Autodesk Inventor part; units mm, degrees
(part 2 of 3)
  line L233 (15.5107, -20.3284) -> (14.1645, -20.3284)
  line L234 (14.1645, -20.3284) -> (14.1645, -19.8987)
  line L235 (14.1645, -19.8987) -> (15.528, -18.3277)
  line L236 (15.528, -18.3277) -> (15.9034, -18.3277)
  line L237 (15.9034, -18.3277) -> (15.9034, -19.9999)
  line L238 (15.9034, -19.9999) -> (16.2665, -19.9999)
  line L239 (16.2665, -19.9999) -> (16.2665, -20.3284)
  line L240 (15.5107, -19.9999) -> (15.5107, -18.8094)
  line L241 (15.5107, -18.8094) -> (14.4856, -19.9999)
  line L242 (14.4856, -19.9999) -> (15.5107, -19.9999)
  line L243 (-27.5269, -31.4126) -> (-26.4993, -28.3646)
  line L244 (-26.4993, -28.3646) -> (-26.0004, -28.3646)
  line L245 (-26.0004, -28.3646) -> (-24.9729, -31.4126)
  line L246 (-24.9729, -31.4126) -> (-25.4002, -31.4126)
  line L247 (-25.4002, -31.4126) -> (-25.6768, -30.5605)
  line L248 (-25.6768, -30.5605) -> (-26.8402, -30.5605)
  line L249 (-26.8402, -30.5605) -> (-27.1168, -31.4126)
  line L250 (-27.1168, -31.4126) -> (-27.5269, -31.4126)
  line L251 (-25.788, -30.2147) -> (-26.2598, -28.7796)
  line L252 (-26.2598, -28.7796) -> (-26.7291, -30.2147)
  line L253 (-26.7291, -30.2147) -> (-25.788, -30.2147)
  line L254 (-22.9178, -31.4126) -> (-23.3031, -31.4126)
  line L255 (-23.3031, -31.4126) -> (-23.3031, -30.1085)
  spline S284 degree 2 poles (-23.3031, -30.1085) (-23.3031, -29.9504) (-23.3328, -29.6787) (-23.3772, -29.5972) knots 0 0 0 1 2 2 2
  spline S285 degree 2 poles (-23.3772, -29.5972) (-23.4242, -29.5107) (-23.5921, -29.4267) (-23.7354, -29.4267) knots 0 0 0 1 2 2 2
  spline S286 degree 2 poles (-23.7354, -29.4267) (-23.8787, -29.4267) (-24.1825, -29.5799) (-24.3282, -29.7034) knots 0 0 0 1 2 2 2
  line L256 (-24.3282, -29.7034) -> (-24.3282, -31.4126)
  line L257 (-24.3282, -31.4126) -> (-24.7135, -31.4126)
  line L258 (-24.7135, -31.4126) -> (-24.7135, -29.1254)
  line L259 (-24.7135, -29.1254) -> (-24.3282, -29.1254)
  line L260 (-24.3282, -29.1254) -> (-24.3282, -29.3798)
  spline S287 degree 2 poles (-24.3282, -29.3798) (-24.1553, -29.2242) (-23.8218, -29.0612) (-23.6341, -29.0612) knots 0 0 0 1 2 2 2
  spline S288 degree 2 poles (-23.6341, -29.0612) (-23.2982, -29.0612) (-22.9178, -29.5058) (-22.9178, -29.9281) knots 0 0 0 1 2 2 2
  line L261 (-22.9178, -29.9281) -> (-22.9178, -31.4126)
  line L262 (-20.6182, -31.4126) -> (-21.0036, -31.4126)
  line L263 (-21.0036, -31.4126) -> (-21.0036, -31.1804)
  spline S289 degree 2 poles (-21.0036, -31.1804) (-21.0925, -31.2545) (-21.2234, -31.3533) (-21.3123, -31.3953) knots 0 0 0 1 2 2 2
  spline S290 degree 2 poles (-21.3123, -31.3953) (-21.3938, -31.4349) (-21.5692, -31.4768) (-21.6853, -31.4768) knots 0 0 0 1 2 2 2
  spline S291 degree 2 poles (-21.6853, -31.4768) (-21.873, -31.4768) (-22.1892, -31.3212) (-22.3003, -31.1706) knots 0 0 0 1 2 2 2
  spline S292 degree 2 poles (-22.3003, -31.1706) (-22.4115, -31.0199) (-22.535, -30.5753) (-22.535, -30.2863) knots 0 0 0 1 2 2 2
  spline S293 degree 2 poles (-22.535, -30.2863) (-22.535, -29.985) (-22.3794, -29.5453) (-22.2435, -29.3798) knots 0 0 0 1 2 2 2
  spline S294 degree 2 poles (-22.2435, -29.3798) (-22.1175, -29.2316) (-21.7643, -29.0612) (-21.5692, -29.0612) knots 0 0 0 1 2 2 2
  spline S295 degree 2 poles (-21.5692, -29.0612) (-21.3988, -29.0612) (-21.1444, -29.1377) (-21.0036, -29.2168) knots 0 0 0 1 2 2 2
  line L264 (-21.0036, -29.2168) -> (-21.0036, -28.2288)
  line L265 (-21.0036, -28.2288) -> (-20.6182, -28.2288)
  line L266 (-20.6182, -28.2288) -> (-20.6182, -31.4126)
  line L267 (-21.0036, -30.8569) -> (-21.0036, -29.5354)
  spline S296 degree 2 poles (-21.0036, -29.5354) (-21.1468, -29.4663) (-21.3741, -29.4144) (-21.505, -29.4144) knots 0 0 0 1 2 2 2
  spline S297 degree 2 poles (-21.505, -29.4144) (-21.8014, -29.4144) (-22.1373, -29.859) (-22.1373, -30.2789) knots 0 0 0 1 2 2 2
  spline S298 degree 2 poles (-22.1373, -30.2789) (-22.1373, -30.684) (-21.8804, -31.1113) (-21.5964, -31.1113) knots 0 0 0 1 2 2 2
  spline S299 degree 2 poles (-21.5964, -31.1113) (-21.4457, -31.1113) (-21.1394, -30.973) (-21.0036, -30.8569) knots 0 0 0 1 2 2 2
  line L268 (-18.8472, -29.5379) -> (-18.867, -29.5379)
  spline S300 degree 2 poles (-18.867, -29.5379) (-18.9115, -29.5255) (-19.0078, -29.5206) (-19.0745, -29.5206) knots 0 0 0 1 2 2 2
  spline S301 degree 2 poles (-19.0745, -29.5206) (-19.2301, -29.5206) (-19.5364, -29.6564) (-19.6747, -29.7898) knots 0 0 0 1 2 2 2
  line L269 (-19.6747, -29.7898) -> (-19.6747, -31.4126)
  line L270 (-19.6747, -31.4126) -> (-20.06, -31.4126)
  line L271 (-20.06, -31.4126) -> (-20.06, -29.1254)
  line L272 (-20.06, -29.1254) -> (-19.6747, -29.1254)
  line L273 (-19.6747, -29.1254) -> (-19.6747, -29.4663)
  spline S302 degree 2 poles (-19.6747, -29.4663) (-19.4647, -29.2785) (-19.151, -29.1254) (-19.0028, -29.1254) knots 0 0 0 1 2 2 2
  spline S303 degree 2 poles (-19.0028, -29.1254) (-18.9436, -29.1254) (-18.8843, -29.1303) (-18.8472, -29.1377) knots 0 0 0 1 2 2 2
  line L274 (-18.8472, -29.1377) -> (-18.8472, -29.5379)
  spline S304 degree 2 poles (-17.5554, -31.4645) (-18.1038, -31.4645) (-18.7064, -30.8495) (-18.7064, -30.2814) knots 0 0 0 1 2 2 2
  spline S305 degree 2 poles (-18.7064, -30.2814) (-18.7064, -29.7231) (-18.1211, -29.0612) (-17.6493, -29.0612) knots 0 0 0 1 2 2 2
  spline S306 degree 2 poles (-17.6493, -29.0612) (-17.4369, -29.0612) (-17.1083, -29.1847) (-16.9873, -29.3156) knots 0 0 0 1 2 2 2
  spline S307 degree 2 poles (-16.9873, -29.3156) (-16.8638, -29.4465) (-16.7329, -29.8244) (-16.7329, -30.0986) knots 0 0 0 1 2 2 2
  line L275 (-16.7329, -30.0986) -> (-16.7329, -30.3085)
  line L276 (-16.7329, -30.3085) -> (-18.3162, -30.3085)
  spline S308 degree 2 poles (-18.3162, -30.3085) (-18.3162, -30.7062) (-17.916, -31.1286) (-17.5604, -31.1286) knots 0 0 0 1 2 2 2
  spline S309 degree 2 poles (-17.5604, -31.1286) (-17.4344, -31.1286) (-17.1899, -31.0718) (-17.0911, -31.0273) knots 0 0 0 1 2 2 2
  spline S310 degree 2 poles (-17.0911, -31.0273) (-16.9873, -30.9779) (-16.8441, -30.8915) (-16.7971, -30.8519) knots 0 0 0 1 2 2 2
  line L277 (-16.7971, -30.8519) -> (-16.7749, -30.8519)
  line L278 (-16.7749, -30.8519) -> (-16.7749, -31.2718)
  spline S311 degree 2 poles (-16.7749, -31.2718) (-16.8416, -31.299) (-17.0441, -31.378) (-17.1232, -31.4003) knots 0 0 0 1 2 2 2
  spline S312 degree 2 poles (-17.1232, -31.4003) (-17.2343, -31.4324) (-17.4171, -31.4645) (-17.5554, -31.4645) knots 0 0 0 1 2 2 2
  spline S313 degree 2 poles (-17.1083, -30.0146) (-17.1133, -29.859) (-17.1775, -29.6317) (-17.2393, -29.5552) knots 0 0 0 1 2 2 2
  spline S314 degree 2 poles (-17.2393, -29.5552) (-17.3059, -29.4687) (-17.5159, -29.3773) (-17.6715, -29.3773) knots 0 0 0 1 2 2 2
  spline S315 degree 2 poles (-17.6715, -29.3773) (-17.8246, -29.3773) (-18.0395, -29.4687) (-18.1285, -29.5576) knots 0 0 0 1 2 2 2
  spline S316 degree 2 poles (-18.1285, -29.5576) (-18.2149, -29.649) (-18.3038, -29.8689) (-18.3162, -30.0146) knots 0 0 0 1 2 2 2
  line L279 (-18.3162, -30.0146) -> (-17.1083, -30.0146)
  line L280 (-13.5713, -29.1254) -> (-14.1517, -31.4126)
  line L281 (-14.1517, -31.4126) -> (-14.5074, -31.4126)
  line L282 (-14.5074, -31.4126) -> (-15.0656, -29.649)
  line L283 (-15.0656, -29.649) -> (-15.6214, -31.4126)
  line L284 (-15.6214, -31.4126) -> (-15.9746, -31.4126)
  line L285 (-15.9746, -31.4126) -> (-16.56, -29.1254)
  line L286 (-16.56, -29.1254) -> (-16.1599, -29.1254)
  line L287 (-16.1599, -29.1254) -> (-15.7548, -30.8964)
  line L288 (-15.7548, -30.8964) -> (-15.2138, -29.1254)
  line L289 (-15.2138, -29.1254) -> (-14.8952, -29.1254)
  line L290 (-14.8952, -29.1254) -> (-14.3395, -30.8964)
  line L291 (-14.3395, -30.8964) -> (-13.9591, -29.1254)
  line L292 (-13.9591, -29.1254) -> (-13.5713, -29.1254)
  line L293 (-10.0713, -28.7253) -> (-11.4891, -28.7253)
  line L294 (-11.4891, -28.7253) -> (-11.4891, -29.5848)
  line L295 (-11.4891, -29.5848) -> (-10.1305, -29.5848)
  line L296 (-10.1305, -29.5848) -> (-10.1305, -29.9454)
  line L297 (-10.1305, -29.9454) -> (-11.4891, -29.9454)
  line L298 (-11.4891, -29.9454) -> (-11.4891, -31.4126)
  line L299 (-11.4891, -31.4126) -> (-11.8941, -31.4126)
  line L300 (-11.8941, -31.4126) -> (-11.8941, -28.3646)
  line L301 (-11.8941, -28.3646) -> (-10.0713, -28.3646)
  line L302 (-10.0713, -28.3646) -> (-10.0713, -28.7253)
  line L303 (-7.9594, -31.4126) -> (-8.3447, -31.4126)
  line L304 (-8.3447, -31.4126) -> (-8.3447, -31.1607)
  spline S317 degree 2 poles (-8.3447, -31.1607) (-8.5226, -31.3163) (-8.8412, -31.4768) (-9.0388, -31.4768) knots 0 0 0 1 2 2 2
  spline S318 degree 2 poles (-9.0388, -31.4768) (-9.187, -31.4768) (-9.4513, -31.378) (-9.5476, -31.2718) knots 0 0 0 1 2 2 2
  spline S319 degree 2 poles (-9.5476, -31.2718) (-9.6464, -31.1656) (-9.7551, -30.8421) (-9.7551, -30.6099) knots 0 0 0 1 2 2 2
  line L305 (-9.7551, -30.6099) -> (-9.7551, -29.1254)
  line L306 (-9.7551, -29.1254) -> (-9.3698, -29.1254)
  line L307 (-9.3698, -29.1254) -> (-9.3698, -30.4296)
  spline S320 degree 2 poles (-9.3698, -30.4296) (-9.3698, -30.6123) (-9.3426, -30.8519) (-9.2957, -30.9409) knots 0 0 0 1 2 2 2
  spline S321 degree 2 poles (-9.2957, -30.9409) (-9.2488, -31.0298) (-9.0882, -31.1113) (-8.9375, -31.1113) knots 0 0 0 1 2 2 2
  spline S322 degree 2 poles (-8.9375, -31.1113) (-8.7967, -31.1113) (-8.4781, -30.9507) (-8.3447, -30.8346) knots 0 0 0 1 2 2 2
  line L308 (-8.3447, -30.8346) -> (-8.3447, -29.1254)
  line L309 (-8.3447, -29.1254) -> (-7.9594, -29.1254)
  line L310 (-7.9594, -29.1254) -> (-7.9594, -31.4126)
  spline S323 degree 2 poles (-7.3197, -31.7782) (-7.2801, -31.7955) (-7.1295, -31.8498) (-7.0331, -31.8721) knots 0 0 0 1 2 2 2
  spline S324 degree 2 poles (-7.0331, -31.8721) (-6.9269, -31.8992) (-6.7466, -31.9313) (-6.6404, -31.9313) knots 0 0 0 1 2 2 2
  spline S325 degree 2 poles (-6.6404, -31.9313) (-6.4626, -31.9313) (-6.2156, -31.8375) (-6.1464, -31.7535) knots 0 0 0 1 2 2 2
  spline S326 degree 2 poles (-6.1464, -31.7535) (-6.0797, -31.6695) (-6.0279, -31.4497) (-6.0279, -31.3089) knots 0 0 0 1 2 2 2
  line L311 (-6.0279, -31.3089) -> (-6.0279, -31.1088)
  spline S327 degree 2 poles (-6.0279, -31.1088) (-6.1835, -31.2447) (-6.4823, -31.3731) (-6.7071, -31.3731) knots 0 0 0 1 2 2 2
  spline S328 degree 2 poles (-6.7071, -31.3731) (-7.0974, -31.3731) (-7.5593, -30.7927) (-7.5593, -30.2468) knots 0 0 0 1 2 2 2
  spline S329 degree 2 poles (-7.5593, -30.2468) (-7.5593, -29.9627) (-7.3987, -29.5231) (-7.2653, -29.3675) knots 0 0 0 1 2 2 2
  spline S330 degree 2 poles (-7.2653, -29.3675) (-7.1369, -29.2217) (-6.7837, -29.0612) (-6.596, -29.0612) knots 0 0 0 1 2 2 2
  spline S331 degree 2 poles (-6.596, -29.0612) (-6.4181, -29.0612) (-6.1588, -29.1452) (-6.0279, -29.2217) knots 0 0 0 1 2 2 2
  line L312 (-6.0279, -29.2217) -> (-6.0056, -29.1254)
  line L313 (-6.0056, -29.1254) -> (-5.6425, -29.1254)
  line L314 (-5.6425, -29.1254) -> (-5.6425, -31.1508)
  spline S332 degree 2 poles (-5.6425, -31.1508) (-5.6425, -31.7337) (-6.1489, -32.2771) (-6.6701, -32.2771) knots 0 0 0 1 2 2 2
  spline S333 degree 2 poles (-6.6701, -32.2771) (-6.838, -32.2771) (-7.1888, -32.2228) (-7.3394, -32.1783) knots 0 0 0 1 2 2 2
  line L315 (-7.3394, -32.1783) -> (-7.3394, -31.7782)
  line L316 (-7.3394, -31.7782) -> (-7.3197, -31.7782)
  line L317 (-6.0279, -30.7927) -> (-6.0279, -29.5354)
  spline S334 degree 2 poles (-6.0279, -29.5354) (-6.1711, -29.4663) (-6.4132, -29.407) (-6.5342, -29.407) knots 0 0 0 1 2 2 2
  spline S335 degree 2 poles (-6.5342, -29.407) (-6.8257, -29.407) (-7.1616, -29.8368) (-7.1616, -30.2394) knots 0 0 0 1 2 2 2
  spline S336 degree 2 poles (-7.1616, -30.2394) (-7.1616, -30.6198) (-6.9072, -31.0174) (-6.6207, -31.0174) knots 0 0 0 1 2 2 2
  spline S337 degree 2 poles (-6.6207, -31.0174) (-6.47, -31.0174) (-6.1538, -30.8989) (-6.0279, -30.7927) knots 0 0 0 1 2 2 2
  spline S338 degree 2 poles (-3.8098, -31.1706) (-3.8567, -31.2051) (-4.0148, -31.3286) (-4.0889, -31.3657) knots 0 0 0 1 2 2 2
  spline S339 degree 2 poles (-4.0889, -31.3657) (-4.1902, -31.42) (-4.3803, -31.4768) (-4.5533, -31.4768) knots 0 0 0 1 2 2 2
  spline S340 degree 2 poles (-4.5533, -31.4768) (-4.694, -31.4768) (-4.9485, -31.3706) (-5.0448, -31.2743) knots 0 0 0 1 2 2 2
  spline S341 degree 2 poles (-5.0448, -31.2743) (-5.1362, -31.1804) (-5.2473, -30.9038) (-5.2473, -30.7507) knots 0 0 0 1 2 2 2
  spline S342 degree 2 poles (-5.2473, -30.7507) (-5.2473, -30.5135) (-5.0473, -30.1776) (-4.8299, -30.0813) knots 0 0 0 1 2 2 2
  spline S343 degree 2 poles (-4.8299, -30.0813) (-4.6372, -29.9924) (-4.1136, -29.9257) (-3.8098, -29.9084) knots 0 0 0 1 2 2 2
  line L318 (-3.8098, -29.9084) -> (-3.8098, -29.8343)
  spline S344 degree 2 poles (-3.8098, -29.8343) (-3.8098, -29.7009) (-3.8913, -29.5354) (-3.9654, -29.4885) knots 0 0 0 1 2 2 2
  spline S345 degree 2 poles (-3.9654, -29.4885) (-4.0395, -29.4416) (-4.2519, -29.4119) (-4.3655, -29.4119) knots 0 0 0 1 2 2 2
  spline S346 degree 2 poles (-4.3655, -29.4119) (-4.4989, -29.4119) (-4.8595, -29.491) (-5.0398, -29.5675) knots 0 0 0 1 2 2 2
  line L319 (-5.0398, -29.5675) -> (-5.0621, -29.5675)
  line L320 (-5.0621, -29.5675) -> (-5.0621, -29.1748)
  spline S347 degree 2 poles (-5.0621, -29.1748) (-4.9559, -29.1452) (-4.5582, -29.0711) (-4.3631, -29.0711) knots 0 0 0 1 2 2 2
  spline S348 degree 2 poles (-4.3631, -29.0711) (-4.1259, -29.0711) (-3.8024, -29.1452) (-3.6739, -29.2415) knots 0 0 0 1 2 2 2
  spline S349 degree 2 poles (-3.6739, -29.2415) (-3.548, -29.3353) (-3.4245, -29.6342) (-3.4245, -29.8491) knots 0 0 0 1 2 2 2
  line L321 (-3.4245, -29.8491) -> (-3.4245, -31.4126)
  line L322 (-3.4245, -31.4126) -> (-3.8098, -31.4126)
  line L323 (-3.8098, -31.4126) -> (-3.8098, -31.1706)
  line L324 (-3.8098, -30.8495) -> (-3.8098, -30.2147)
  spline S350 degree 2 poles (-3.8098, -30.2147) (-3.9481, -30.227) (-4.3655, -30.269) (-4.4964, -30.3085) knots 0 0 0 1 2 2 2
  spline S351 degree 2 poles (-4.4964, -30.3085) (-4.6496, -30.3555) (-4.8497, -30.5506) (-4.8497, -30.7235) knots 0 0 0 1 2 2 2
  spline S352 degree 2 poles (-4.8497, -30.7235) (-4.8497, -30.9211) (-4.6274, -31.1212) (-4.4149, -31.1212) knots 0 0 0 1 2 2 2
  spline S353 degree 2 poles (-4.4149, -31.1212) (-4.2346, -31.1212) (-3.9382, -30.9656) (-3.8098, -30.8495) knots 0 0 0 1 2 2 2
  spline S354 degree 2 poles (-2.1919, -31.4571) (-2.5056, -31.4571) (-2.8588, -31.0989) (-2.8588, -30.7111) knots 0 0 0 1 2 2 2
  line L325 (-2.8588, -30.7111) -> (-2.8588, -29.444)
  line L326 (-2.8588, -29.444) -> (-3.1182, -29.444)
  line L327 (-3.1182, -29.444) -> (-3.1182, -29.1254)
  line L328 (-3.1182, -29.1254) -> (-2.8588, -29.1254)
  line L329 (-2.8588, -29.1254) -> (-2.8588, -28.4684)
  line L330 (-2.8588, -28.4684) -> (-2.4735, -28.4684)
  line L331 (-2.4735, -28.4684) -> (-2.4735, -29.1254)
  line L332 (-2.4735, -29.1254) -> (-1.7646, -29.1254)
  line L333 (-1.7646, -29.1254) -> (-1.7646, -29.444)
  line L334 (-1.7646, -29.444) -> (-2.4735, -29.444)
  line L335 (-2.4735, -29.444) -> (-2.4735, -30.5333)
  spline S355 degree 2 poles (-2.4735, -30.5333) (-2.4735, -30.7062) (-2.4611, -30.8964) (-2.4192, -30.9779) knots 0 0 0 1 2 2 2
  spline S356 degree 2 poles (-2.4192, -30.9779) (-2.3846, -31.0495) (-2.229, -31.1212) (-2.0956, -31.1212) knots 0 0 0 1 2 2 2
  spline S357 degree 2 poles (-2.0956, -31.1212) (-2.0017, -31.1212) (-1.8264, -31.0644) (-1.7868, -31.0471) knots 0 0 0 1 2 2 2
  line L336 (-1.7868, -31.0471) -> (-1.7646, -31.0471)
  line L337 (-1.7646, -31.0471) -> (-1.7646, -31.3929)
  spline S358 degree 2 poles (-1.7646, -31.3929) (-1.8733, -31.4225) (-2.0956, -31.4571) (-2.1919, -31.4571) knots 0 0 0 1 2 2 2
  spline S359 degree 2 poles (-0.4876, -31.4645) (-1.0359, -31.4645) (-1.6386, -30.8495) (-1.6386, -30.2814) knots 0 0 0 1 2 2 2
  spline S360 degree 2 poles (-1.6386, -30.2814) (-1.6386, -29.7231) (-1.0532, -29.0612) (-0.5815, -29.0612) knots 0 0 0 1 2 2 2
  spline S361 degree 2 poles (-0.5815, -29.0612) (-0.369, -29.0612) (-0.0405, -29.1847) (0.0805, -29.3156) knots 0 0 0 1 2 2 2
  spline S362 degree 2 poles (0.0805, -29.3156) (0.204, -29.4465) (0.3349, -29.8244) (0.3349, -30.0986) knots 0 0 0 1 2 2 2
  line L338 (0.3349, -30.0986) -> (0.3349, -30.3085)
  line L339 (0.3349, -30.3085) -> (-1.2484, -30.3085)
  spline S363 degree 2 poles (-1.2484, -30.3085) (-1.2484, -30.7062) (-0.8482, -31.1286) (-0.4925, -31.1286) knots 0 0 0 1 2 2 2
  spline S364 degree 2 poles (-0.4925, -31.1286) (-0.3666, -31.1286) (-0.122, -31.0718) (-0.0232, -31.0273) knots 0 0 0 1 2 2 2
  spline S365 degree 2 poles (-0.0232, -31.0273) (0.0805, -30.9779) (0.2238, -30.8915) (0.2707, -30.8519) knots 0 0 0 1 2 2 2
  line L340 (0.2707, -30.8519) -> (0.2929, -30.8519)
  line L341 (0.2929, -30.8519) -> (0.2929, -31.2718)
  spline S366 degree 2 poles (0.2929, -31.2718) (0.2262, -31.299) (0.0237, -31.378) (-0.0554, -31.4003) knots 0 0 0 1 2 2 2
  spline S367 degree 2 poles (-0.0554, -31.4003) (-0.1665, -31.4324) (-0.3493, -31.4645) (-0.4876, -31.4645) knots 0 0 0 1 2 2 2
  spline S368 degree 2 poles (-0.0405, -30.0146) (-0.0455, -29.859) (-0.1097, -29.6317) (-0.1714, -29.5552) knots 0 0 0 1 2 2 2
  spline S369 degree 2 poles (-0.1714, -29.5552) (-0.2381, -29.4687) (-0.4481, -29.3773) (-0.6037, -29.3773) knots 0 0 0 1 2 2 2
  spline S370 degree 2 poles (-0.6037, -29.3773) (-0.7568, -29.3773) (-0.9717, -29.4687) (-1.0606, -29.5576) knots 0 0 0 1 2 2 2
  spline S371 degree 2 poles (-1.0606, -29.5576) (-1.1471, -29.649) (-1.236, -29.8689) (-1.2484, -30.0146) knots 0 0 0 1 2 2 2
  line L342 (-1.2484, -30.0146) -> (-0.0405, -30.0146)
  line L343 (3.0939, -30.2641) -> (1.9404, -30.2641)
  line L344 (1.9404, -30.2641) -> (1.9404, -29.8936)
  line L345 (1.9404, -29.8936) -> (3.0939, -29.8936)
  line L346 (3.0939, -29.8936) -> (3.0939, -30.2641)
  line L347 (4.566, -31.4126) -> (5.5936, -28.3646)
  line L348 (5.5936, -28.3646) -> (6.0925, -28.3646)
  line L349 (6.0925, -28.3646) -> (7.12, -31.4126)
  line L350 (7.12, -31.4126) -> (6.6927, -31.4126)
  line L351 (6.6927, -31.4126) -> (6.4161, -30.5605)
  line L352 (6.4161, -30.5605) -> (5.2527, -30.5605)
  line L353 (5.2527, -30.5605) -> (4.9761, -31.4126)
  line L354 (4.9761, -31.4126) -> (4.566, -31.4126)
  line L355 (6.3049, -30.2147) -> (5.8332, -28.7796)
  line L356 (5.8332, -28.7796) -> (5.3639, -30.2147)
  line L357 (5.3639, -30.2147) -> (6.3049, -30.2147)
  line L358 (7.7721, -31.4126) -> (7.3868, -31.4126)
  line L359 (7.3868, -31.4126) -> (7.3868, -28.2288)
  line L360 (7.3868, -28.2288) -> (7.7721, -28.2288)
  line L361 (7.7721, -28.2288) -> (7.7721, -31.4126)
  spline S372 degree 2 poles (9.3307, -31.4645) (8.7824, -31.4645) (8.1797, -30.8495) (8.1797, -30.2814) knots 0 0 0 1 2 2 2
  spline S373 degree 2 poles (8.1797, -30.2814) (8.1797, -29.7231) (8.7651, -29.0612) (9.2368, -29.0612) knots 0 0 0 1 2 2 2
  spline S374 degree 2 poles (9.2368, -29.0612) (9.4493, -29.0612) (9.7778, -29.1847) (9.8988, -29.3156) knots 0 0 0 1 2 2 2
  spline S375 degree 2 poles (9.8988, -29.3156) (10.0223, -29.4465) (10.1532, -29.8244) (10.1532, -30.0986) knots 0 0 0 1 2 2 2
  line L362 (10.1532, -30.0986) -> (10.1532, -30.3085)
  line L363 (10.1532, -30.3085) -> (8.5699, -30.3085)
  spline S376 degree 2 poles (8.5699, -30.3085) (8.5699, -30.7062) (8.9701, -31.1286) (9.3258, -31.1286) knots 0 0 0 1 2 2 2
  spline S377 degree 2 poles (9.3258, -31.1286) (9.4517, -31.1286) (9.6963, -31.0718) (9.7951, -31.0273) knots 0 0 0 1 2 2 2
  spline S378 degree 2 poles (9.7951, -31.0273) (9.8988, -30.9779) (10.0421, -30.8915) (10.089, -30.8519) knots 0 0 0 1 2 2 2
  line L364 (10.089, -30.8519) -> (10.1112, -30.8519)
  line L365 (10.1112, -30.8519) -> (10.1112, -31.2718)
  spline S379 degree 2 poles (10.1112, -31.2718) (10.0445, -31.299) (9.842, -31.378) (9.763, -31.4003) knots 0 0 0 1 2 2 2
  spline S380 degree 2 poles (9.763, -31.4003) (9.6518, -31.4324) (9.469, -31.4645) (9.3307, -31.4645) knots 0 0 0 1 2 2 2
  spline S381 degree 2 poles (9.7778, -30.0146) (9.7728, -29.859) (9.7086, -29.6317) (9.6469, -29.5552) knots 0 0 0 1 2 2 2
  spline S382 degree 2 poles (9.6469, -29.5552) (9.5802, -29.4687) (9.3702, -29.3773) (9.2146, -29.3773) knots 0 0 0 1 2 2 2
  spline S383 degree 2 poles (9.2146, -29.3773) (9.0615, -29.3773) (8.8466, -29.4687) (8.7577, -29.5576) knots 0 0 0 1 2 2 2
  spline S384 degree 2 poles (8.7577, -29.5576) (8.6712, -29.649) (8.5823, -29.8689) (8.5699, -30.0146) knots 0 0 0 1 2 2 2
  line L366 (8.5699, -30.0146) -> (9.7778, -30.0146)
  spline S385 degree 2 poles (11.4525, -31.4645) (11.2153, -31.4645) (10.8226, -31.3188) (10.6818, -31.1706) knots 0 0 0 1 2 2 2
  spline S386 degree 2 poles (10.6818, -31.1706) (10.541, -31.0248) (10.3854, -30.5753) (10.3854, -30.274) knots 0 0 0 1 2 2 2
  spline S387 degree 2 poles (10.3854, -30.274) (10.3854, -29.9726) (10.546, -29.5329) (10.6818, -29.3847) knots 0 0 0 1 2 2 2
  spline S388 degree 2 poles (10.6818, -29.3847) (10.8177, -29.2341) (11.2203, -29.0735) (11.4525, -29.0735) knots 0 0 0 1 2 2 2
  spline S389 degree 2 poles (11.4525, -29.0735) (11.6402, -29.0735) (11.9909, -29.1797) (12.1268, -29.2489) knots 0 0 0 1 2 2 2
  line L367 (12.1268, -29.2489) -> (12.1268, -29.6811)
  line L368 (12.1268, -29.6811) -> (12.1045, -29.6811)
  spline S390 degree 2 poles (12.1045, -29.6811) (12.0625, -29.6466) (11.9341, -29.5576) (11.8427, -29.5107) knots 0 0 0 1 2 2 2
  spline S391 degree 2 poles (11.8427, -29.5107) (11.7612, -29.4712) (11.5438, -29.4094) (11.445, -29.4094) knots 0 0 0 1 2 2 2
  spline S392 degree 2 poles (11.445, -29.4094) (11.1462, -29.4094) (10.7831, -29.8615) (10.7831, -30.274) knots 0 0 0 1 2 2 2
  spline S393 degree 2 poles (10.7831, -30.274) (10.7831, -30.6766) (11.1338, -31.1286) (11.445, -31.1286) knots 0 0 0 1 2 2 2
  spline S394 degree 2 poles (11.445, -31.1286) (11.6328, -31.1286) (11.9736, -30.973) (12.1045, -30.8519) knots 0 0 0 1 2 2 2
  line L369 (12.1045, -30.8519) -> (12.1268, -30.8519)
  line L370 (12.1268, -30.8519) -> (12.1268, -31.2842)
  spline S395 degree 2 poles (12.1268, -31.2842) (12.07, -31.3114) (11.8971, -31.3879) (11.8279, -31.4052) knots 0 0 0 1 2 2 2
  spline S396 degree 2 poles (11.8279, -31.4052) (11.7291, -31.4349) (11.5735, -31.4645) (11.4525, -31.4645) knots 0 0 0 1 2 2 2
  spline S397 degree 2 poles (16.2196, -29.8911) (16.2196, -30.3085) (15.8812, -30.9804) (15.5971, -31.1681) knots 0 0 0 1 2 2 2
  spline S398 degree 2 poles (15.5971, -31.1681) (15.365, -31.3138) (14.8882, -31.4126) (14.5177, -31.4126) knots 0 0 0 1 2 2 2
  line L371 (14.5177, -31.4126) -> (13.8163, -31.4126)
  line L372 (13.8163, -31.4126) -> (13.8163, -28.3646)
  line L373 (13.8163, -28.3646) -> (14.5103, -28.3646)
  spline S399 degree 2 poles (14.5103, -28.3646) (14.9401, -28.3646) (15.4292, -28.4931) (15.6021, -28.6067) knots 0 0 0 1 2 2 2
  spline S400 degree 2 poles (15.6021, -28.6067) (15.896, -28.8018) (16.2196, -29.4465) (16.2196, -29.8911) knots 0 0 0 1 2 2 2
  spline S401 degree 2 poles (15.7972, -29.8862) (15.7972, -29.5354) (15.565, -29.0389) (15.3353, -28.8982) knots 0 0 0 1 2 2 2
  spline S402 degree 2 poles (15.3353, -28.8982) (15.1723, -28.8018) (14.8043, -28.7154) (14.5301, -28.7154) knots 0 0 0 1 2 2 2
  line L374 (14.5301, -28.7154) -> (14.2213, -28.7154)
  line L375 (14.2213, -28.7154) -> (14.2213, -31.0619)
  line L376 (14.2213, -31.0619) -> (14.5301, -31.0619)
  spline S403 degree 2 poles (14.5301, -31.0619) (14.7993, -31.0619) (15.2069, -30.9754) (15.3724, -30.8593) knots 0 0 0 1 2 2 2
  spline S404 degree 2 poles (15.3724, -30.8593) (15.5848, -30.7161) (15.7972, -30.2418) (15.7972, -29.8862) knots 0 0 0 1 2 2 2
  spline S405 degree 2 poles (17.9041, -31.1706) (17.8572, -31.2051) (17.6991, -31.3286) (17.625, -31.3657) knots 0 0 0 1 2 2 2
  spline S406 degree 2 poles (17.625, -31.3657) (17.5238, -31.42) (17.3336, -31.4768) (17.1607, -31.4768) knots 0 0 0 1 2 2 2
  spline S407 degree 2 poles (17.1607, -31.4768) (17.0199, -31.4768) (16.7655, -31.3706) (16.6691, -31.2743) knots 0 0 0 1 2 2 2
  spline S408 degree 2 poles (16.6691, -31.2743) (16.5777, -31.1804) (16.4666, -30.9038) (16.4666, -30.7507) knots 0 0 0 1 2 2 2
  spline S409 degree 2 poles (16.4666, -30.7507) (16.4666, -30.5135) (16.6667, -30.1776) (16.884, -30.0813) knots 0 0 0 1 2 2 2
  spline S410 degree 2 poles (16.884, -30.0813) (17.0767, -29.9924) (17.6003, -29.9257) (17.9041, -29.9084) knots 0 0 0 1 2 2 2
  line L377 (17.9041, -29.9084) -> (17.9041, -29.8343)
  spline S411 degree 2 poles (17.9041, -29.8343) (17.9041, -29.7009) (17.8226, -29.5354) (17.7485, -29.4885) knots 0 0 0 1 2 2 2
  spline S412 degree 2 poles (17.7485, -29.4885) (17.6744, -29.4416) (17.462, -29.4119) (17.3484, -29.4119) knots 0 0 0 1 2 2 2
  spline S413 degree 2 poles (17.3484, -29.4119) (17.215, -29.4119) (16.8544, -29.491) (16.6741, -29.5675) knots 0 0 0 1 2 2 2
  line L378 (16.6741, -29.5675) -> (16.6518, -29.5675)
  line L379 (16.6518, -29.5675) -> (16.6518, -29.1748)
  spline S414 degree 2 poles (16.6518, -29.1748) (16.758, -29.1452) (17.1557, -29.0711) (17.3509, -29.0711) knots 0 0 0 1 2 2 2
  spline S415 degree 2 poles (17.3509, -29.0711) (17.588, -29.0711) (17.9115, -29.1452) (18.04, -29.2415) knots 0 0 0 1 2 2 2
  spline S416 degree 2 poles (18.04, -29.2415) (18.166, -29.3353) (18.2895, -29.6342) (18.2895, -29.8491) knots 0 0 0 1 2 2 2
  line L380 (18.2895, -29.8491) -> (18.2895, -31.4126)
  line L381 (18.2895, -31.4126) -> (17.9041, -31.4126)
  line L382 (17.9041, -31.4126) -> (17.9041, -31.1706)
  line L383 (17.9041, -30.8495) -> (17.9041, -30.2147)
  spline S417 degree 2 poles (17.9041, -30.2147) (17.7658, -30.227) (17.3484, -30.269) (17.2175, -30.3085) knots 0 0 0 1 2 2 2
  spline S418 degree 2 poles (17.2175, -30.3085) (17.0643, -30.3555) (16.8643, -30.5506) (16.8643, -30.7235) knots 0 0 0 1 2 2 2
  spline S419 degree 2 poles (16.8643, -30.7235) (16.8643, -30.9211) (17.0866, -31.1212) (17.299, -31.1212) knots 0 0 0 1 2 2 2
  spline S420 degree 2 poles (17.299, -31.1212) (17.4793, -31.1212) (17.7757, -30.9656) (17.9041, -30.8495) knots 0 0 0 1 2 2 2
  line L384 (21.4239, -31.4126) -> (21.4239, -30.0887)
  spline S421 degree 2 poles (21.4239, -30.0887) (21.4239, -29.9306) (21.3992, -29.6614) (21.3597, -29.5873) knots 0 0 0 1 2 2 2
  spline S422 degree 2 poles (21.3597, -29.5873) (21.3202, -29.5058) (21.1695, -29.4267) (21.0386, -29.4267) knots 0 0 0 1 2 2 2
  spline S423 degree 2 poles (21.0386, -29.4267) (20.92, -29.4267) (20.6483, -29.5725) (20.5051, -29.7108) knots 0 0 0 1 2 2 2
  spline S424 degree 2 poles (20.5051, -29.7108) (20.5075, -29.7454) (20.5125, -29.8417) (20.5125, -29.9059) knots 0 0 0 1 2 2 2
  line L385 (20.5125, -29.9059) -> (20.5125, -31.4126)
  line L386 (20.5125, -31.4126) -> (20.1272, -31.4126)
  line L387 (20.1272, -31.4126) -> (20.1272, -30.0887)
  spline S425 degree 2 poles (20.1272, -30.0887) (20.1272, -29.9306) (20.1025, -29.6614) (20.0629, -29.5873) knots 0 0 0 1 2 2 2
  spline S426 degree 2 poles (20.0629, -29.5873) (20.0234, -29.5058) (19.8727, -29.4267) (19.7418, -29.4267) knots 0 0 0 1 2 2 2
  spline S427 degree 2 poles (19.7418, -29.4267) (19.6183, -29.4267) (19.3442, -29.5823) (19.2157, -29.7034) knots 0 0 0 1 2 2 2
  line L388 (19.2157, -29.7034) -> (19.2157, -31.4126)
  line L389 (19.2157, -31.4126) -> (18.8304, -31.4126)
  line L390 (18.8304, -31.4126) -> (18.8304, -29.1254)
  line L391 (18.8304, -29.1254) -> (19.2157, -29.1254)
  line L392 (19.2157, -29.1254) -> (19.2157, -29.3773)
  spline S428 degree 2 poles (19.2157, -29.3773) (19.3664, -29.2267) (19.6628, -29.0612) (19.8406, -29.0612) knots 0 0 0 1 2 2 2
  spline S429 degree 2 poles (19.8406, -29.0612) (20.0432, -29.0612) (20.3569, -29.2464) (20.4384, -29.4564) knots 0 0 0 1 2 2 2
  spline S430 degree 2 poles (20.4384, -29.4564) (20.6137, -29.2612) (20.9447, -29.0612) (21.1374, -29.0612) knots 0 0 0 1 2 2 2
  spline S431 degree 2 poles (21.1374, -29.0612) (21.2856, -29.0612) (21.5277, -29.1526) (21.6166, -29.2563) knots 0 0 0 1 2 2 2
  spline S432 degree 2 poles (21.6166, -29.2563) (21.708, -29.36) (21.8092, -29.6713) (21.8092, -29.9059) knots 0 0 0 1 2 2 2
  line L393 (21.8092, -29.9059) -> (21.8092, -31.4126)
  line L394 (21.8092, -31.4126) -> (21.4239, -31.4126)
  line L395 (22.7429, -31.4126) -> (22.3576, -31.4126)
  line L396 (22.3576, -31.4126) -> (22.3576, -29.1254)
  line L397 (22.3576, -29.1254) -> (22.7429, -29.1254)
  line L398 (22.7429, -29.1254) -> (22.7429, -31.4126)
  line L399 (22.7701, -28.745) -> (22.3329, -28.745)
  line L400 (22.3329, -28.745) -> (22.3329, -28.3449)
  line L401 (22.3329, -28.3449) -> (22.7701, -28.3449)
  line L402 (22.7701, -28.3449) -> (22.7701, -28.745)
  spline S433 degree 2 poles (24.3015, -31.4645) (23.7531, -31.4645) (23.1505, -30.8495) (23.1505, -30.2814) knots 0 0 0 1 2 2 2
  spline S434 degree 2 poles (23.1505, -30.2814) (23.1505, -29.7231) (23.7358, -29.0612) (24.2076, -29.0612) knots 0 0 0 1 2 2 2
  spline S435 degree 2 poles (24.2076, -29.0612) (24.42, -29.0612) (24.7486, -29.1847) (24.8696, -29.3156) knots 0 0 0 1 2 2 2
  spline S436 degree 2 poles (24.8696, -29.3156) (24.9931, -29.4465) (25.124, -29.8244) (25.124, -30.0986) knots 0 0 0 1 2 2 2
  line L403 (25.124, -30.0986) -> (25.124, -30.3085)
  line L404 (25.124, -30.3085) -> (23.5407, -30.3085)
  spline S437 degree 2 poles (23.5407, -30.3085) (23.5407, -30.7062) (23.9409, -31.1286) (24.2965, -31.1286) knots 0 0 0 1 2 2 2
  spline S438 degree 2 poles (24.2965, -31.1286) (24.4225, -31.1286) (24.667, -31.0718) (24.7658, -31.0273) knots 0 0 0 1 2 2 2
  spline S439 degree 2 poles (24.7658, -31.0273) (24.8696, -30.9779) (25.0128, -30.8915) (25.0598, -30.8519) knots 0 0 0 1 2 2 2
  line L405 (25.0598, -30.8519) -> (25.082, -30.8519)
  line L406 (25.082, -30.8519) -> (25.082, -31.2718)
  spline S440 degree 2 poles (25.082, -31.2718) (25.0153, -31.299) (24.8128, -31.378) (24.7337, -31.4003) knots 0 0 0 1 2 2 2
  spline S441 degree 2 poles (24.7337, -31.4003) (24.6226, -31.4324) (24.4398, -31.4645) (24.3015, -31.4645) knots 0 0 0 1 2 2 2
  spline S442 degree 2 poles (24.7486, -30.0146) (24.7436, -29.859) (24.6794, -29.6317) (24.6176, -29.5552) knots 0 0 0 1 2 2 2
  spline S443 degree 2 poles (24.6176, -29.5552) (24.551, -29.4687) (24.341, -29.3773) (24.1854, -29.3773) knots 0 0 0 1 2 2 2
  spline S444 degree 2 poles (24.1854, -29.3773) (24.0322, -29.3773) (23.8174, -29.4687) (23.7284, -29.5576) knots 0 0 0 1 2 2 2
  spline S445 degree 2 poles (23.7284, -29.5576) (23.642, -29.649) (23.5531, -29.8689) (23.5407, -30.0146) knots 0 0 0 1 2 2 2
  line L407 (23.5407, -30.0146) -> (24.7486, -30.0146)
  line L408 (27.31, -31.4126) -> (26.9246, -31.4126)
  line L409 (26.9246, -31.4126) -> (26.9246, -30.1085)
  spline S446 degree 2 poles (26.9246, -30.1085) (26.9246, -29.9504) (26.895, -29.6787) (26.8505, -29.5972) knots 0 0 0 1 2 2 2
  spline S447 degree 2 poles (26.8505, -29.5972) (26.8036, -29.5107) (26.6356, -29.4267) (26.4924, -29.4267) knots 0 0 0 1 2 2 2
  spline S448 degree 2 poles (26.4924, -29.4267) (26.3491, -29.4267) (26.0453, -29.5799) (25.8996, -29.7034) knots 0 0 0 1 2 2 2
  line L410 (25.8996, -29.7034) -> (25.8996, -31.4126)
  line L411 (25.8996, -31.4126) -> (25.5143, -31.4126)
  line L412 (25.5143, -31.4126) -> (25.5143, -29.1254)
  line L413 (25.5143, -29.1254) -> (25.8996, -29.1254)
  line L414 (25.8996, -29.1254) -> (25.8996, -29.3798)
  spline S449 degree 2 poles (25.8996, -29.3798) (26.0725, -29.2242) (26.4059, -29.0612) (26.5937, -29.0612) knots 0 0 0 1 2 2 2
  spline S450 degree 2 poles (26.5937, -29.0612) (26.9296, -29.0612) (27.31, -29.5058) (27.31, -29.9281) knots 0 0 0 1 2 2 2
  line L415 (27.31, -29.9281) -> (27.31, -31.4126)
  line L416 (-24.406, -33.3831) -> (-25.436, -35.0825)
  line L417 (-25.436, -35.0825) -> (-25.436, -36.4311)
  line L418 (-25.436, -36.4311) -> (-25.8411, -36.4311)
  line L419 (-25.8411, -36.4311) -> (-25.8411, -35.1244)
  line L420 (-25.8411, -35.1244) -> (-26.8711, -33.3831)
  line L421 (-26.8711, -33.3831) -> (-26.4215, -33.3831)
  line L422 (-26.4215, -33.3831) -> (-25.6361, -34.7243)
  line L423 (-25.6361, -34.7243) -> (-24.8358, -33.3831)
  line L424 (-24.8358, -33.3831) -> (-24.406, -33.3831)
  line L425 (-22.3584, -34.1438) -> (-23.2204, -36.4311)
  line L426 (-23.2204, -36.4311) -> (-23.5662, -36.4311)
  line L427 (-23.5662, -36.4311) -> (-24.4208, -34.1438)
  line L428 (-24.4208, -34.1438) -> (-24.0034, -34.1438)
  line L429 (-24.0034, -34.1438) -> (-23.3785, -35.905)
  line L430 (-23.3785, -35.905) -> (-22.7585, -34.1438)
  line L431 (-22.7585, -34.1438) -> (-22.3584, -34.1438)
  spline S451 degree 2 poles (-20.7924, -36.189) (-20.8393, -36.2236) (-20.9974, -36.3471) (-21.0715, -36.3841) knots 0 0 0 1 2 2 2
  spline S452 degree 2 poles (-21.0715, -36.3841) (-21.1728, -36.4385) (-21.3629, -36.4953) (-21.5358, -36.4953) knots 0 0 0 1 2 2 2
  spline S453 degree 2 poles (-21.5358, -36.4953) (-21.6766, -36.4953) (-21.9311, -36.3891) (-22.0274, -36.2928) knots 0 0 0 1 2 2 2
  spline S454 degree 2 poles (-22.0274, -36.2928) (-22.1188, -36.1989) (-22.2299, -35.9223) (-22.2299, -35.7691) knots 0 0 0 1 2 2 2
  spline S455 degree 2 poles (-22.2299, -35.7691) (-22.2299, -35.532) (-22.0299, -35.1961) (-21.8125, -35.0997) knots 0 0 0 1 2 2 2
  spline S456 degree 2 poles (-21.8125, -35.0997) (-21.6198, -35.0108) (-21.0962, -34.9441) (-20.7924, -34.9268) knots 0 0 0 1 2 2 2
  line L432 (-20.7924, -34.9268) -> (-20.7924, -34.8527)
  spline S457 degree 2 poles (-20.7924, -34.8527) (-20.7924, -34.7194) (-20.8739, -34.5539) (-20.948, -34.5069) knots 0 0 0 1 2 2 2
  spline S458 degree 2 poles (-20.948, -34.5069) (-21.0221, -34.46) (-21.2345, -34.4304) (-21.3481, -34.4304) knots 0 0 0 1 2 2 2
  spline S459 degree 2 poles (-21.3481, -34.4304) (-21.4815, -34.4304) (-21.8421, -34.5094) (-22.0224, -34.586) knots 0 0 0 1 2 2 2
  line L433 (-22.0224, -34.586) -> (-22.0447, -34.586)
  line L434 (-22.0447, -34.586) -> (-22.0447, -34.1932)
  spline S460 degree 2 poles (-22.0447, -34.1932) (-21.9385, -34.1636) (-21.5408, -34.0895) (-21.3457, -34.0895) knots 0 0 0 1 2 2 2
  spline S461 degree 2 poles (-21.3457, -34.0895) (-21.1085, -34.0895) (-20.785, -34.1636) (-20.6565, -34.2599) knots 0 0 0 1 2 2 2
  spline S462 degree 2 poles (-20.6565, -34.2599) (-20.5306, -34.3538) (-20.4071, -34.6527) (-20.4071, -34.8676) knots 0 0 0 1 2 2 2
  line L435 (-20.4071, -34.8676) -> (-20.4071, -36.4311)
  line L436 (-20.4071, -36.4311) -> (-20.7924, -36.4311)
  line L437 (-20.7924, -36.4311) -> (-20.7924, -36.189)
  line L438 (-20.7924, -35.8679) -> (-20.7924, -35.2331)
  spline S463 degree 2 poles (-20.7924, -35.2331) (-20.9307, -35.2455) (-21.3481, -35.2875) (-21.479, -35.327) knots 0 0 0 1 2 2 2
  spline S464 degree 2 poles (-21.479, -35.327) (-21.6322, -35.3739) (-21.8322, -35.569) (-21.8322, -35.7419) knots 0 0 0 1 2 2 2
  spline S465 degree 2 poles (-21.8322, -35.7419) (-21.8322, -35.9395) (-21.6099, -36.1396) (-21.3975, -36.1396) knots 0 0 0 1 2 2 2
  spline S466 degree 2 poles (-21.3975, -36.1396) (-21.2172, -36.1396) (-20.9208, -35.984) (-20.7924, -35.8679) knots 0 0 0 1 2 2 2
  line L439 (-18.0704, -36.4311) -> (-18.4557, -36.4311)
  line L440 (-18.4557, -36.4311) -> (-18.4557, -35.1269)
  spline S467 degree 2 poles (-18.4557, -35.1269) (-18.4557, -34.9688) (-18.4854, -34.6971) (-18.5298, -34.6156) knots 0 0 0 1 2 2 2
  spline S468 degree 2 poles (-18.5298, -34.6156) (-18.5768, -34.5292) (-18.7447, -34.4452) (-18.888, -34.4452) knots 0 0 0 1 2 2 2
  spline S469 degree 2 poles (-18.888, -34.4452) (-19.0313, -34.4452) (-19.3351, -34.5983) (-19.4808, -34.7218) knots 0 0 0 1 2 2 2
  line L441 (-19.4808, -34.7218) -> (-19.4808, -36.4311)
  line L442 (-19.4808, -36.4311) -> (-19.8661, -36.4311)
  line L443 (-19.8661, -36.4311) -> (-19.8661, -34.1438)
  line L444 (-19.8661, -34.1438) -> (-19.4808, -34.1438)
  line L445 (-19.4808, -34.1438) -> (-19.4808, -34.3983)
  spline S470 degree 2 poles (-19.4808, -34.3983) (-19.3079, -34.2426) (-18.9744, -34.0796) (-18.7867, -34.0796) knots 0 0 0 1 2 2 2
  spline S471 degree 2 poles (-18.7867, -34.0796) (-18.4508, -34.0796) (-18.0704, -34.5242) (-18.0704, -34.9466) knots 0 0 0 1 2 2 2
  line L446 (-18.0704, -34.9466) -> (-18.0704, -36.4311)
  spline S472 degree 2 poles (-14.2641, -34.3019) (-14.2641, -34.4995) (-14.4049, -34.8552) (-14.5309, -34.9787) knots 0 0 0 1 2 2 2
  spline S473 degree 2 poles (-14.5309, -34.9787) (-14.689, -35.1343) (-15.1163, -35.2949) (-15.4423, -35.2949) knots 0 0 0 1 2 2 2
  line L447 (-15.4423, -35.2949) -> (-15.7856, -35.2949)
  line L448 (-15.7856, -35.2949) -> (-15.7856, -36.4311)
  line L449 (-15.7856, -36.4311) -> (-16.1907, -36.4311)
  line L450 (-16.1907, -36.4311) -> (-16.1907, -33.3831)
  line L451 (-16.1907, -33.3831) -> (-15.425, -33.3831)
  spline S474 degree 2 poles (-15.425, -33.3831) (-15.1533, -33.3831) (-14.7729, -33.472) (-14.6272, -33.5733) knots 0 0 0 1 2 2 2
  spline S475 degree 2 poles (-14.6272, -33.5733) (-14.4568, -33.6894) (-14.2641, -34.0475) (-14.2641, -34.3019) knots 0 0 0 1 2 2 2
  spline S476 degree 2 poles (-14.6865, -34.3143) (-14.6865, -34.1562) (-14.7952, -33.924) (-14.9063, -33.8499) knots 0 0 0 1 2 2 2
  spline S477 degree 2 poles (-14.9063, -33.8499) (-15.0027, -33.7857) (-15.2595, -33.7338) (-15.4497, -33.7338) knots 0 0 0 1 2 2 2
  line L452 (-15.4497, -33.7338) -> (-15.7856, -33.7338)
  line L453 (-15.7856, -33.7338) -> (-15.7856, -34.9491)
  line L454 (-15.7856, -34.9491) -> (-15.509, -34.9491)
  spline S478 degree 2 poles (-15.509, -34.9491) (-15.262, -34.9491) (-14.9582, -34.87) (-14.8594, -34.7663) knots 0 0 0 1 2 2 2
  spline S479 degree 2 poles (-14.8594, -34.7663) (-14.768, -34.6749) (-14.6865, -34.46) (-14.6865, -34.3143) knots 0 0 0 1 2 2 2
  line L455 (-13.5157, -36.4311) -> (-13.901, -36.4311)
  line L456 (-13.901, -36.4311) -> (-13.901, -34.1438)
  line L457 (-13.901, -34.1438) -> (-13.5157, -34.1438)
  line L458 (-13.5157, -34.1438) -> (-13.5157, -36.4311)
  line L459 (-13.4885, -33.7635) -> (-13.9257, -33.7635)
  line L460 (-13.9257, -33.7635) -> (-13.9257, -33.3633)
  line L461 (-13.9257, -33.3633) -> (-13.4885, -33.3633)
  line L462 (-13.4885, -33.3633) -> (-13.4885, -33.7635)
  spline S480 degree 2 poles (-11.9571, -36.483) (-12.5055, -36.483) (-13.1082, -35.8679) (-13.1082, -35.2998) knots 0 0 0 1 2 2 2
  spline S481 degree 2 poles (-13.1082, -35.2998) (-13.1082, -34.7416) (-12.5228, -34.0796) (-12.051, -34.0796) knots 0 0 0 1 2 2 2
  spline S482 degree 2 poles (-12.051, -34.0796) (-11.8386, -34.0796) (-11.5101, -34.2031) (-11.389, -34.334) knots 0 0 0 1 2 2 2
  spline S483 degree 2 poles (-11.389, -34.334) (-11.2655, -34.4649) (-11.1346, -34.8429) (-11.1346, -35.117) knots 0 0 0 1 2 2 2
  line L463 (-11.1346, -35.117) -> (-11.1346, -35.327)
  line L464 (-11.1346, -35.327) -> (-12.7179, -35.327)
  spline S484 degree 2 poles (-12.7179, -35.327) (-12.7179, -35.7247) (-12.3177, -36.147) (-11.9621, -36.147) knots 0 0 0 1 2 2 2
  spline S485 degree 2 poles (-11.9621, -36.147) (-11.8361, -36.147) (-11.5916, -36.0902) (-11.4928, -36.0458) knots 0 0 0 1 2 2 2
  spline S486 degree 2 poles (-11.4928, -36.0458) (-11.389, -35.9964) (-11.2458, -35.9099) (-11.1988, -35.8704) knots 0 0 0 1 2 2 2
  line L465 (-11.1988, -35.8704) -> (-11.1766, -35.8704)
  line L466 (-11.1766, -35.8704) -> (-11.1766, -36.2903)
  spline S487 degree 2 poles (-11.1766, -36.2903) (-11.2433, -36.3175) (-11.4458, -36.3965) (-11.5249, -36.4187) knots 0 0 0 1 2 2 2
  spline S488 degree 2 poles (-11.5249, -36.4187) (-11.636, -36.4508) (-11.8188, -36.483) (-11.9571, -36.483) knots 0 0 0 1 2 2 2
  spline S489 degree 2 poles (-11.5101, -35.0331) (-11.515, -34.8774) (-11.5792, -34.6502) (-11.641, -34.5736) knots 0 0 0 1 2 2 2
  spline S490 degree 2 poles (-11.641, -34.5736) (-11.7077, -34.4872) (-11.9176, -34.3958) (-12.0732, -34.3958) knots 0 0 0 1 2 2 2
  spline S491 degree 2 poles (-12.0732, -34.3958) (-12.2264, -34.3958) (-12.4412, -34.4872) (-12.5302, -34.5761) knots 0 0 0 1 2 2 2
  spline S492 degree 2 poles (-12.5302, -34.5761) (-12.6166, -34.6675) (-12.7055, -34.8873) (-12.7179, -35.0331) knots 0 0 0 1 2 2 2
  line L467 (-12.7179, -35.0331) -> (-11.5101, -35.0331)
  line L468 (-9.5316, -34.5563) -> (-9.5513, -34.5563)
  spline S493 degree 2 poles (-9.5513, -34.5563) (-9.5958, -34.544) (-9.6921, -34.539) (-9.7588, -34.539) knots 0 0 0 1 2 2 2
  spline S494 degree 2 poles (-9.7588, -34.539) (-9.9144, -34.539) (-10.2207, -34.6749) (-10.359, -34.8083) knots 0 0 0 1 2 2 2
  line L469 (-10.359, -34.8083) -> (-10.359, -36.4311)
  line L470 (-10.359, -36.4311) -> (-10.7443, -36.4311)
  line L471 (-10.7443, -36.4311) -> (-10.7443, -34.1438)
  line L472 (-10.7443, -34.1438) -> (-10.359, -34.1438)
  line L473 (-10.359, -34.1438) -> (-10.359, -34.4847)
  spline S495 degree 2 poles (-10.359, -34.4847) (-10.1491, -34.297) (-9.8354, -34.1438) (-9.6872, -34.1438) knots 0 0 0 1 2 2 2
  spline S496 degree 2 poles (-9.6872, -34.1438) (-9.6279, -34.1438) (-9.5686, -34.1488) (-9.5316, -34.1562) knots 0 0 0 1 2 2 2
  line L474 (-9.5316, -34.1562) -> (-9.5316, -34.5563)
  line L475 (-8.0199, -34.5563) -> (-8.0397, -34.5563)
  spline S497 degree 2 poles (-8.0397, -34.5563) (-8.0841, -34.544) (-8.1805, -34.539) (-8.2472, -34.539) knots 0 0 0 1 2 2 2
  spline S498 degree 2 poles (-8.2472, -34.539) (-8.4028, -34.539) (-8.7091, -34.6749) (-8.8474, -34.8083) knots 0 0 0 1 2 2 2
  line L476 (-8.8474, -34.8083) -> (-8.8474, -36.4311)
  line L477 (-8.8474, -36.4311) -> (-9.2327, -36.4311)
  line L478 (-9.2327, -36.4311) -> (-9.2327, -34.1438)
  line L479 (-9.2327, -34.1438) -> (-8.8474, -34.1438)
  line L480 (-8.8474, -34.1438) -> (-8.8474, -34.4847)
  spline S499 degree 2 poles (-8.8474, -34.4847) (-8.6374, -34.297) (-8.3237, -34.1438) (-8.1755, -34.1438) knots 0 0 0 1 2 2 2
  spline S500 degree 2 poles (-8.1755, -34.1438) (-8.1162, -34.1438) (-8.057, -34.1488) (-8.0199, -34.1562) knots 0 0 0 1 2 2 2
  line L481 (-8.0199, -34.1562) -> (-8.0199, -34.5563)
  spline S501 degree 2 poles (-6.7281, -36.483) (-7.2764, -36.483) (-7.8791, -35.8679) (-7.8791, -35.2998) knots 0 0 0 1 2 2 2
  spline S502 degree 2 poles (-7.8791, -35.2998) (-7.8791, -34.7416) (-7.2937, -34.0796) (-6.822, -34.0796) knots 0 0 0 1 2 2 2
  spline S503 degree 2 poles (-6.822, -34.0796) (-6.6095, -34.0796) (-6.281, -34.2031) (-6.16, -34.334) knots 0 0 0 1 2 2 2
  spline S504 degree 2 poles (-6.16, -34.334) (-6.0365, -34.4649) (-5.9056, -34.8429) (-5.9056, -35.117) knots 0 0 0 1 2 2 2
  line L482 (-5.9056, -35.117) -> (-5.9056, -35.327)
  line L483 (-5.9056, -35.327) -> (-7.4889, -35.327)
  spline S505 degree 2 poles (-7.4889, -35.327) (-7.4889, -35.7247) (-7.0887, -36.147) (-6.733, -36.147) knots 0 0 0 1 2 2 2
  spline S506 degree 2 poles (-6.733, -36.147) (-6.6071, -36.147) (-6.3625, -36.0902) (-6.2637, -36.0458) knots 0 0 0 1 2 2 2
  spline S507 degree 2 poles (-6.2637, -36.0458) (-6.16, -35.9964) (-6.0167, -35.9099) (-5.9698, -35.8704) knots 0 0 0 1 2 2 2
  line L484 (-5.9698, -35.8704) -> (-5.9476, -35.8704)
  line L485 (-5.9476, -35.8704) -> (-5.9476, -36.2903)
  spline S508 degree 2 poles (-5.9476, -36.2903) (-6.0143, -36.3175) (-6.2168, -36.3965) (-6.2958, -36.4187) knots 0 0 0 1 2 2 2
  spline S509 degree 2 poles (-6.2958, -36.4187) (-6.407, -36.4508) (-6.5898, -36.483) (-6.7281, -36.483) knots 0 0 0 1 2 2 2
  spline S510 degree 2 poles (-6.281, -35.0331) (-6.286, -34.8774) (-6.3502, -34.6502) (-6.4119, -34.5736) knots 0 0 0 1 2 2 2
  spline S511 degree 2 poles (-6.4119, -34.5736) (-6.4786, -34.4872) (-6.6886, -34.3958) (-6.8442, -34.3958) knots 0 0 0 1 2 2 2
  spline S512 degree 2 poles (-6.8442, -34.3958) (-6.9973, -34.3958) (-7.2122, -34.4872) (-7.3011, -34.5761) knots 0 0 0 1 2 2 2
  spline S513 degree 2 poles (-7.3011, -34.5761) (-7.3876, -34.6675) (-7.4765, -34.8873) (-7.4889, -35.0331) knots 0 0 0 1 2 2 2
  line L486 (-7.4889, -35.0331) -> (-6.281, -35.0331)
  spline S514 degree 2 poles (-3.028, -35.6382) (-3.028, -36.0383) (-3.5171, -36.4731) (-3.9296, -36.4731) knots 0 0 0 1 2 2 2
  spline S515 degree 2 poles (-3.9296, -36.4731) (-4.0284, -36.4731) (-4.3569, -36.4385) (-4.468, -36.4138) knots 0 0 0 1 2 2 2
  line L487 (-4.468, -36.4138) -> (-4.468, -36.0235)
  line L488 (-4.468, -36.0235) -> (-4.4458, -36.0235)
  spline S516 degree 2 poles (-4.4458, -36.0235) (-4.3618, -36.0532) (-4.1124, -36.1223) (-3.9839, -36.1223) knots 0 0 0 1 2 2 2
  spline S517 degree 2 poles (-3.9839, -36.1223) (-3.7962, -36.1223) (-3.5714, -36.0359) (-3.5195, -35.9568) knots 0 0 0 1 2 2 2
  spline S518 degree 2 poles (-3.5195, -35.9568) (-3.4627, -35.8753) (-3.4331, -35.6382) (-3.4331, -35.4826) knots 0 0 0 1 2 2 2
  line L489 (-3.4331, -35.4826) -> (-3.4331, -33.7067)
  line L490 (-3.4331, -33.7067) -> (-4.0778, -33.7067)
  line L491 (-4.0778, -33.7067) -> (-4.0778, -33.3831)
  line L492 (-4.0778, -33.3831) -> (-3.028, -33.3831)
  line L493 (-3.028, -33.3831) -> (-3.028, -35.6382)
  line L494 (-1.2471, -34.5563) -> (-1.2669, -34.5563)
  spline S519 degree 2 poles (-1.2669, -34.5563) (-1.3114, -34.544) (-1.4077, -34.539) (-1.4744, -34.539) knots 0 0 0 1 2 2 2
  spline S520 degree 2 poles (-1.4744, -34.539) (-1.63, -34.539) (-1.9363, -34.6749) (-2.0746, -34.8083) knots 0 0 0 1 2 2 2
  line L495 (-2.0746, -34.8083) -> (-2.0746, -36.4311)
  line L496 (-2.0746, -36.4311) -> (-2.4599, -36.4311)
  line L497 (-2.4599, -36.4311) -> (-2.4599, -34.1438)
  line L498 (-2.4599, -34.1438) -> (-2.0746, -34.1438)
  line L499 (-2.0746, -34.1438) -> (-2.0746, -34.4847)
  spline S521 degree 2 poles (-2.0746, -34.4847) (-1.8646, -34.297) (-1.5509, -34.1438) (-1.4027, -34.1438) knots 0 0 0 1 2 2 2
  spline S522 degree 2 poles (-1.4027, -34.1438) (-1.3435, -34.1438) (-1.2842, -34.1488) (-1.2471, -34.1562) knots 0 0 0 1 2 2 2
  line L500 (-1.2471, -34.1562) -> (-1.2471, -34.5563)
  line L501 (-0.3505, -36.4311) -> (-0.8396, -36.4311)
  line L502 (-0.8396, -36.4311) -> (-0.8396, -35.8482)
  line L503 (-0.8396, -35.8482) -> (-0.3505, -35.8482)
  line L504 (-0.3505, -35.8482) -> (-0.3505, -36.4311)
  line L505 (2.6901, -35.2825) -> (1.5366, -35.2825)
  line L506 (1.5366, -35.2825) -> (1.5366, -34.912)
  line L507 (1.5366, -34.912) -> (2.6901, -34.912)
  line L508 (2.6901, -34.912) -> (2.6901, -35.2825)
  line L509 (4.4907, -36.4311) -> (4.4907, -33.3831)
  line L510 (4.4907, -33.3831) -> (6.3976, -33.3831)
  line L511 (6.3976, -33.3831) -> (6.3976, -33.7437)
  line L512 (6.3976, -33.7437) -> (4.8958, -33.7437)
  line L513 (4.8958, -33.7437) -> (4.8958, -34.5786)
  line L514 (4.8958, -34.5786) -> (6.2963, -34.5786)
  line L515 (6.2963, -34.5786) -> (6.2963, -34.9392)
  line L516 (6.2963, -34.9392) -> (4.8958, -34.9392)
  line L517 (4.8958, -34.9392) -> (4.8958, -36.0705)
  line L518 (4.8958, -36.0705) -> (6.3976, -36.0705)
  line L519 (6.3976, -36.0705) -> (6.3976, -36.4311)
  line L520 (6.3976, -36.4311) -> (4.4907, -36.4311)
  line L521 (8.0253, -34.5563) -> (8.0055, -34.5563)
  spline S523 degree 2 poles (8.0055, -34.5563) (7.9611, -34.544) (7.8648, -34.539) (7.7981, -34.539) knots 0 0 0 1 2 2 2
  spline S524 degree 2 poles (7.7981, -34.539) (7.6425, -34.539) (7.3362, -34.6749) (7.1979, -34.8083) knots 0 0 0 1 2 2 2
  line L522 (7.1979, -34.8083) -> (7.1979, -36.4311)
  line L523 (7.1979, -36.4311) -> (6.8125, -36.4311)
  line L524 (6.8125, -36.4311) -> (6.8125, -34.1438)
  line L525 (6.8125, -34.1438) -> (7.1979, -34.1438)
  line L526 (7.1979, -34.1438) -> (7.1979, -34.4847)
  spline S525 degree 2 poles (7.1979, -34.4847) (7.4078, -34.297) (7.7215, -34.1438) (7.8697, -34.1438) knots 0 0 0 1 2 2 2
  spline S526 degree 2 poles (7.8697, -34.1438) (7.929, -34.1438) (7.9883, -34.1488) (8.0253, -34.1562) knots 0 0 0 1 2 2 2
  line L527 (8.0253, -34.1562) -> (8.0253, -34.5563)
  line L528 (8.7169, -36.4311) -> (8.3316, -36.4311)
  line L529 (8.3316, -36.4311) -> (8.3316, -34.1438)
  line L530 (8.3316, -34.1438) -> (8.7169, -34.1438)
  line L531 (8.7169, -34.1438) -> (8.7169, -36.4311)
  line L532 (8.7441, -33.7635) -> (8.3069, -33.7635)
  line L533 (8.3069, -33.7635) -> (8.3069, -33.3633)
  line L534 (8.3069, -33.3633) -> (8.7441, -33.3633)
  line L535 (8.7441, -33.3633) -> (8.7441, -33.7635)
  line L536 (11.177, -36.4311) -> (10.6707, -36.4311)
  line L537 (10.6707, -36.4311) -> (9.821, -35.327)
  line L538 (9.821, -35.327) -> (9.6679, -35.4752)
  line L539 (9.6679, -35.4752) -> (9.6679, -36.4311)
  line L540 (9.6679, -36.4311) -> (9.2825, -36.4311)
  line L541 (9.2825, -36.4311) -> (9.2825, -33.2472)
  line L542 (9.2825, -33.2472) -> (9.6679, -33.2472)
  line L543 (9.6679, -33.2472) -> (9.6679, -35.1096)
  line L544 (9.6679, -35.1096) -> (10.5719, -34.1438)
  line L545 (10.5719, -34.1438) -> (11.0511, -34.1438)
  line L546 (11.0511, -34.1438) -> (10.1125, -35.0997)
  line L547 (10.1125, -35.0997) -> (11.177, -36.4311)
  spline S527 degree 2 poles (14.7759, -35.4949) (14.7759, -35.7222) (14.603, -36.0705) (14.4597, -36.1841) knots 0 0 0 1 2 2 2
  spline S528 degree 2 poles (14.4597, -36.1841) (14.2868, -36.3175) (13.8941, -36.4311) (13.5828, -36.4311) knots 0 0 0 1 2 2 2
  line L548 (13.5828, -36.4311) -> (12.7085, -36.4311)
  line L549 (12.7085, -36.4311) -> (12.7085, -33.3831)
  line L550 (12.7085, -33.3831) -> (13.5162, -33.3831)
  spline S529 degree 2 poles (13.5162, -33.3831) (13.8422, -33.3831) (14.1682, -33.4251) (14.3164, -33.5066) knots 0 0 0 1 2 2 2
  spline S530 degree 2 poles (14.3164, -33.5066) (14.4819, -33.593) (14.6326, -33.8771) (14.6326, -34.0697) knots 0 0 0 1 2 2 2
  spline S531 degree 2 poles (14.6326, -34.0697) (14.6326, -34.2846) (14.4054, -34.6255) (14.2053, -34.7218) knots 0 0 0 1 2 2 2
  line L551 (14.2053, -34.7218) -> (14.2053, -34.7366)
  spline S532 degree 2 poles (14.2053, -34.7366) (14.477, -34.8107) (14.7759, -35.2035) (14.7759, -35.4949) knots 0 0 0 1 2 2 2
  spline S533 degree 2 poles (14.3535, -35.5122) (14.3535, -35.3393) (14.2547, -35.117) (14.1065, -35.038) knots 0 0 0 1 2 2 2